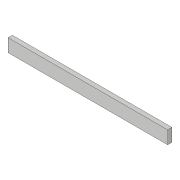
# Autodesk Inventor part: line_edge_parkinglot_2_1
Saved by Autodesk Inventor 2018 (Build 220112000, 112)
## iProperties
Created: 2017-11-13
Part Number: line_edge_parkinglot_2_1
Material: Generic
Document SubType Name: Modeling
Designer: Platform
Density: 1 g/cm^3
Appearance: Default
Author: Platform
Autodesk Inventor part; units mm, degrees
ref_plane "YZ Plane" through (0, 0, 0) normal (1, 0, 0) x (0, 1, 0)
ref_plane "XZ Plane" through (0, 0, 0) normal (0, 1, 0) x (-1, 0, 0)
ref_plane "XY Plane" through (0, 0, 0) normal (0, 0, 1) x (1, 0, 0)
sketch "Sketch1" plane through (0, 0, 0) normal (0, 0, 1) x (1, 0, 0)
  line L0 (0, 0) -> (0, 15)
  line L1 (0, 0) -> (15, 0) construction
  line L2 (0, 15) -> (185, 15)
  line L3 (185, 15) -> (185, 0)
  line L4 (185, 0) -> (0, 0)
  dimension "d0" = 15
  dimension "d1" = 90
  dimension "d2" = 185
  dimension "d3" = 90
  dimension "d4" = 15
  dimension "d5" = 90
  constraints: 10 end point, 3 perpendicular, 1 horizontal, 1 vertical
  measures "d0" distance of L0.start L0.end
  measures "d1" angle of L1 L0
  measures "d2" distance of L0.end L2.end
  measures "d3" angle of L0 L2
  measures "d4" distance of L2.end L3.end
  measures "d5" angle of L2 L3
extrude "Extrusion1" add sketch "Sketch1" along normal blind 5
body "Solid1"
